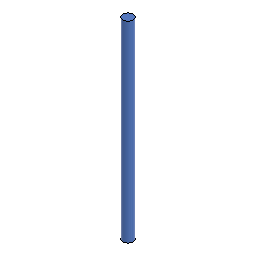
Final Pure Assembly (Autodesk Fusion 360 archive; units mm, degrees)
design "FPA_Guiding Rod"
Autodesk Fusion 360 part; units mm, degrees
(part 1 of 2)
sketch "Sketch2" plane through (0, 0, 0) normal (0, 0, 1) x (1, 0, 0)
  circle A0 centre (0, 0) radius 4
  dimension "d2" = 8
  constraint coincident A0.centre origin
  measures "d2" diameter of A0
extrude "Extrude1" add sketch "Sketch2" along normal blind 150 in component "8mm Diameter Guiding Rod"
component "8mm Diameter Guiding Rod" placed x (1, 0, 0) y (0, 1, 0) z (0, 0, 1) at (0, 0, 0)
equation "length = 150 mm"
equation "d4 = length"

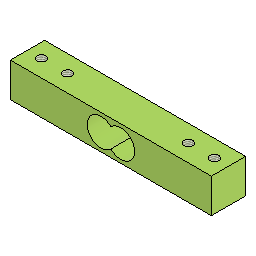
design "FPA_Load Cell"
Autodesk Fusion 360 part; units mm, degrees
sketch "Sketch1" plane through (0, 0, 0) normal (1, 0, 0) x (0, 1, 0)
  line L0 (0, 0) -> (12.8, 0)
  line L1 (12.8, 0) -> (12.8, 12.8)
  line L2 (12.8, 12.8) -> (0, 12.8)
  line L3 (0, 12.8) -> (0, 0)
  dimension "d1" = 12.8
  dimension "d2" = 12.8
  constraint horizontal L0
  constraint vertical L1
  constraint horizontal L2
  constraint vertical L3
  constraint coincident L0.start L3.end
  measures "d1" distance of L0.start L0.end
  measures "d2" distance of L0.start L2.end
extrude "Extrude1" add sketch "Sketch1" along normal blind 75.1 in component "Load Cell"
sketch "Sketch2" plane through (0, 0, 0) normal (0, -1, 0) x (1, 0, 0)
  line L0 (0, 12.8) -> (0, 0)
  line L1 (0, 0) -> (75.1, 0)
  line L2 (75.1, 0) -> (75.1, 12.8)
  line L3 (75.1, 12.8) -> (0, 12.8)
  line L4 (0, 6.4) -> (75.1, 6.4) construction
  line L5 (75.1, 6.4) -> (46.4, 6.4) construction
  circle A0 centre (41.25, 6.4) radius 5.15
  line L6 (37.55, 0) -> (37.55, 12.8) construction
  circle A1 centre (33.85, 6.4) radius 5.15
  point P0 (37.55, 9.9822)
  point P1 (37.55, 2.8178)
  point P2 (28.7, 6.4)
  dimension "d5" = 28.7
  dimension "d6" = 10.3
  dimension "d7" = 7.1645
  dimension "d8" = 28.7
  constraint midpoint L0 L4.start
  constraint midpoint L2 L4.end
  constraint coincident L4 L5.end
  constraint coincident L4 A0.centre
  constraint coincident L5.end A0
  constraint midpoint L1 L6.start
  constraint midpoint L3 L6.end
  constraint symmetric A0 L6 A1
  constraint coincident L6 P0
  constraint coincident A1 P0
  constraint coincident A1 P1
  constraint coincident A0 P1
  constraint coincident A1 P2
  constraint coincident L4 P2
  measures "d5" distance of L4.end L5.end
  measures "d6" diameter of A0
  measures "d7" distance of P0 P1
  measures "d8" distance of L4.start P2
extrude "Extrude2" cut sketch "Sketch2" against normal blind 12.8 contours A0 A1 | A0 A1 | A0 A1 in component "Load Cell"
sketch "Sketch3" plane through (0, 0, 12.8) normal (0, 0, 1) x (-1, 0, 0)
  line L0 (0, -12.8) -> (0, 0)
  line L1 (0, 0) -> (-75.1, 0)
  line L2 (-75.1, 0) -> (-75.1, -12.8)
  line L3 (-75.1, -12.8) -> (0, -12.8)
  line L4 (-75.1, -6.4) -> (0, -6.4) construction
  line L5 (-75.1, -6.4) -> (-71.5, -6.4) construction
  circle A0 centre (-69.834, -6.4) radius 1.666
  circle A1 centre (-60.102, -6.4) radius 1.666
  line L6 (-37.55, -12.8) -> (-37.55, 0) construction
  circle A2 centre (-14.998, -6.4) radius 1.666
  circle A3 centre (-5.266, -6.4) radius 1.666
  point P0 (-71.5, -6.4)
  point P1 (-61.768, -6.4)
  point P2 (-68.168, -6.4)
  dimension "d11" = 3.6
  dimension "d25" = 3.332
  dimension "d26" = 6.4
  constraint midpoint L2 L4.start
  constraint midpoint L0 L4.end
  constraint perpendicular L2 L5
  constraint coincident L4 A0.centre
  constraint coincident A0 P0
  constraint coincident L4 P0
  constraint coincident P0 L5.end
  constraint coincident L4 A1.centre
  constraint equal A0 A1
  constraint coincident A1 P1
  constraint coincident L4 P1
  constraint coincident A0 P2
  constraint coincident L4 P2
  constraint midpoint L3 L6.start
  constraint midpoint L1 L6.end
  constraint symmetric A0 L6 A3
  constraint symmetric A1 L6 A2
  measures "d11" distance of L4.start P0
  measures "d25" diameter of A0
  measures "d26" distance of P1 P2
hole "Hole3" at (5.266, 6.4, 12.8) at (14.998, 6.4, 12.8) at (60.102, 6.4, 12.8) at (69.834, 6.4, 12.8) direction (0, 0, -1) diameter 3.332 depth 16 tip angle 118 in component "Load Cell"
thread "Thread3" "ISO Metric profile 4.0 M4x0.7 M4x0.7 6H" thread offset 0 thread depth 7.4 in component "Load Cell"
component "Load Cell" placed x (1, 0, 0) y (0, 1, 0) z (0, 0, 1) at (0, 0, 0)

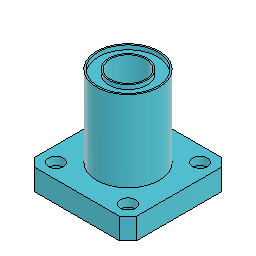
design "FPA_ Linear Bearing Square Flange"
Autodesk Fusion 360 part; units mm, degrees
sketch "Sketch1" plane through (0, 0, 0) normal (0, 0, 1) x (1, 0, 0)
  circle A0 centre (0, 0) radius 4
  circle A1 centre (0, 0) radius 7.5
  line L0 (12, -12) -> (-12, -12)
  line L1 (-12, -12) -> (-12, 12)
  line L2 (-12, 12) -> (12, 12)
  line L3 (12, 12) -> (12, -12)
  line L4 (12, -12) -> (-12, 12) construction
  line L5 (-12, -12) -> (12, 12) construction
  circle A2 centre (0, 0) radius 12 construction
  circle A3 centre (8.4853, 8.4853) radius 1.75
  circle A4 centre (8.4853, 8.4853) radius 3
  circle A5 centre (-8.4853, 8.4853) radius 3
  circle A6 centre (-8.4853, 8.4853) radius 1.75
  circle A7 centre (-8.4853, -8.4853) radius 3
  circle A8 centre (-8.4853, -8.4853) radius 1.75
  circle A9 centre (8.4853, -8.4853) radius 3
  circle A10 centre (8.4853, -8.4853) radius 1.75
  dimension "d1" = 8
  dimension "d2" = 15
  dimension "d3" = 24
  dimension "d4" = 24
  dimension "d5" = 24
  dimension "d8" = 3.5
  dimension "d9" = 6
  dimension "d11" = 360
  constraint coincident A0.centre A1.centre
  constraint horizontal L0
  constraint perpendicular L0 L1
  constraint parallel L0 L2
  constraint parallel L1 L3
  constraint coincident L4 A0.centre
  constraint coincident L5 A0.centre
  constraint concentric A0 A2
  constraint coincident L5 A3.centre
  constraint coincident A2 A3.centre
  constraint concentric A3 A4
  measures "d1" diameter of A0
  measures "d2" diameter of A1
  measures "d3" distance of L1.end L2.end
  measures "d4" distance of L0.end L1.end
  measures "d5" diameter of A2
  measures "d8" diameter of A3
  measures "d9" diameter of A4
extrude "Extrude1" add sketch "Sketch1" against normal blind 5 contours A0 | A1 | L0 L1 L2 L3 | A3 | A4 | A5 | A6 | A7 | A8 | A9 | A10 in component "Component"
extrude "Extrude2" cut sketch "Sketch1" against normal blind 1.9 contours A3 | A6 | A8 | A10 in component "Component"
sketch "Sketch2" plane through (0, 0, -5) normal (0, 0, -1) x (1, 0, 0)
  line L0 (-12, -12) -> (12, -12)
  line L1 (12, -12) -> (12, 12)
  line L2 (12, 12) -> (-12, 12)
  line L3 (-12, 12) -> (-12, -12)
  circle A0 centre (8.4853, 8.4853) radius 3
  circle A1 centre (8.4853, -8.4853) radius 3
  circle A2 centre (-8.4853, -8.4853) radius 3
  circle A3 centre (-8.4853, 8.4853) radius 3
extrude "Extrude3" cut sketch "Sketch2" against normal blind 3.1 contours A0 | A1 | A2 | A3 in component "Component"
extrude "Extrude4" add sketch "Sketch1" along normal blind 19 contours A1 in component "Component"
sketch "Sketch3" plane through (0, 0, 19) normal (0, 0, 1) x (-1, 0, 0)
  circle A0 centre (0, 0) radius 4
  circle A1 centre (0, 0) radius 7.5
  circle A2 centre (0, 0) radius 4
  circle A3 centre (0, 0) radius 7.5
  circle A4 centre (0, 0) radius 4.5
  circle A5 centre (0, 0) radius 7
  dimension "d18" = 0.5
  dimension "d19" = -0.5
extrude "Extrude5" cut sketch "Sketch3" against normal blind 1 contours A5 in component "Component"
extrude "Extrude6" cut 1 faces at (-1.2456, 0.0132, 0) along direction (0, 0, -1) blind 5 in component "Component"
sketch "Sketch4" plane through (0, 0, -5) normal (0, 0, -1) x (1, 0, 0)
  line L0 (12, -12) -> (12, 12)
  line L1 (12, 12) -> (-12, 12)
  line L2 (-12, 12) -> (-12, -12)
  line L3 (-12, -12) -> (12, -12)
  circle A0 centre (0, 0) radius 4
  circle A1 centre (-8.4853, -8.4853) radius 3
  circle A2 centre (8.4853, -8.4853) radius 3
  circle A3 centre (-8.4853, 8.4853) radius 3
  circle A4 centre (8.4853, 8.4853) radius 3
  circle A5 centre (0, 0) radius 4.5
  circle A6 centre (0, 0) radius 4
  circle A7 centre (0, 0) radius 7
  circle A8 centre (0, 0) radius 7.5
extrude "Extrude7" cut sketch "Sketch4" against normal blind 1 contours A7 in component "Component"
move_face "OffsetFaces1" offset -0.15 1 faces at (3.995, -0.1994, 11) in component "Component"
chamfer "Chamfer2" distance 2 angle 45 4 edges at (-12, -12, -2.5) (-12, 12, -2.5) (12, -12, -2.5) (12, 12, -2.5) in component "Component"
move_face "OffsetFaces2" offset -0.15 1 faces at (7.4907, 0.3738, 6.3333) in component "Component"
component "Component" placed x (1, 0, 0) y (0, 1, 0) z (0, 0, 1) at (0, 0, 0)

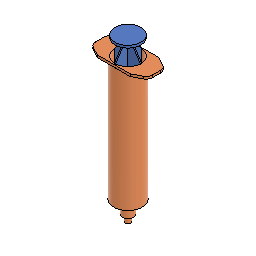
design "FPA_20ml Luer Lock Syringe"
Autodesk Fusion 360 part; units mm, degrees
sketch "Sketch1" plane through (0, 0, 0) normal (0, 1, 0) x (1, 0, 0)
  line L0 (0, 0) -> (11.155, 0)
  line L1 (11.155, 0) -> (11.155, -115) construction
  line L2 (11.155, 0) -> (11.155, -95)
  line L3 (11.155, -95) -> (11.155, -101.75) construction
  line L4 (11.155, -101.75) -> (11.155, -110) construction
  line L5 (11.155, -95) -> (4.4407, -96.7991)
  line L6 (11.155, -95) -> (0, -95) construction
  line L7 (4.4407, -96.7991) -> (4.4407, -105.0848)
  line L8 (4.4407, -105.0848) -> (2.2202, -105.0848)
  line L9 (2.2202, -105.0848) -> (2.2202, -110.0848)
  line L10 (0, -110.0848) -> (2.2202, -110.0848)
  line L11 (0, 0) -> (0, -110.0848)
  dimension "d1" = 11.155
  dimension "d3" = 95
  dimension "d4" = 6.75
  dimension "d5" = 8.25
  dimension "d6" = 165
  dimension "d7" = 2.2205
  dimension "d8" = 8.2857
  dimension "d9" = 5
  dimension "d10" = 2.2202
  dimension "d66" = 115
  dimension "d67" = 110.0848
  constraint coincident L0.start L11.start
  constraint horizontal L0
  constraint perpendicular L0 L1
  constraint perpendicular L0 L2
  constraint parallel L1 L3
  constraint parallel L1 L4
  constraint horizontal L6
  constraint parallel L4 L7
  constraint perpendicular L1 L8
  constraint perpendicular L8 L9
  constraint vertical L11
  constraint perpendicular L10 L11
  constraint coincident L6.end L11
  measures "d1" distance of L0.start L0.end
  measures "d3" distance of L0.end L2.end
  measures "d4" distance of L2.end L3.end
  measures "d5" distance of L3.end L4.end
  measures "d6" angle of L5 L6
  measures "d7" distance of L7.end L8.end
  measures "d8" distance of L5.end L7.end
  measures "d9" distance of L8.end L9.end
  measures "d10" distance of L9.end L10.start
  measures "d66" distance of L0.end L1.end
  measures "d67" distance of L0.start L10.start
revolve "Revolve1" add sketch "Sketch1" angle 360 about axis through (0, 0, 0) along (0, 0, 1) makes body 1 in component "30ml Luer Lock Barrel"
shell "Shell1" thickness 1 removed faces 1 at (-1.6561, 2.7028, 0) on bodies 1 in component "30ml Luer Lock Barrel"
sketch "Sketch2" plane through (0, 0, 110.0848) normal (0, 0, 1) x (-1, 0, 0)
  circle A0 centre (0, 0) radius 2.2202
  circle A1 centre (0, 0) radius 1.2202
extrude "Extrude1" cut sketch "Sketch2" against normal blind 6.86 contours A1 bodies 1 in component "30ml Luer Lock Barrel"
sketch "Sketch3" plane through (0, 0, 0) normal (0, 0, -1) x (1, 0, 0)
  circle A0 centre (0, 0) radius 10.155
  circle A1 centre (0, 0) radius 11.155
  line L0 (22.35, -11.155) -> (-22.35, -11.155)
  line L1 (-22.35, -11.155) -> (-22.35, 11.155)
  line L2 (-22.35, 11.155) -> (22.35, 11.155)
  line L3 (22.35, 11.155) -> (22.35, -11.155)
  line L4 (22.35, -11.155) -> (-22.35, 11.155) construction
  line L5 (-22.35, -11.155) -> (22.35, 11.155) construction
  circle A2 centre (0, 0) radius 10.155
  dimension "d15" = 44.7
  dimension "d16" = 22.31
  constraint horizontal L0
  constraint perpendicular L0 L1
  constraint parallel L0 L2
  constraint parallel L1 L3
  constraint coincident L4 A0.centre
  constraint coincident L5 A0.centre
  constraint coincident A0.centre A1.centre
  measures "d15" distance of L1.end L2.end
  measures "d16" distance of L0.end L1.end
extrude "Extrude2" add sketch "Sketch3" along normal blind 1.86 bodies 1 in component "30ml Luer Lock Barrel"
chamfer "Chamfer1" distance 5 distance2 9.5 2 edges at (22.35, -11.155, -0.93) (-22.35, 11.155, -0.93) measured on face at (22.35, -3.7183, -0.62) measured on face at (-22.35, 3.7183, -0.62) tangent chain off on bodies 1 in component "30ml Luer Lock Barrel"
chamfer "Chamfer1" distance 9.5 distance2 5 2 edges at (22.35, 11.155, -0.93) (-22.35, -11.155, -0.93) measured on face at (0, 11.155, -1.24) measured on face at (0, -11.155, -1.24) tangent chain off on bodies 1 in component "30ml Luer Lock Barrel"
fillet "Fillet1" radius 5 4 edges at (22.35, -6.155, -0.93) (22.35, 6.155, -0.93) (-22.35, -6.155, -0.93) (-22.35, 6.155, -0.93) on bodies 1 in component "30ml Luer Lock Barrel"
sketch "Sketch4" plane through (0, 0, 0) normal (0, 1, 0) x (1, 0, 0)
  line L0 (-11.155, -95) -> (11.155, -95)
  line L1 (-4.4407, -96.7991) -> (4.4407, -96.7991)
  line L2 (-4.4407, -96.7991) -> (-11.155, -95)
  line L3 (-11.155, -95) -> (11.155, -95)
  line L4 (11.155, -95) -> (4.4407, -96.7991)
  line L5 (-4.4407, -96.7991) -> (0, -97.989)
  line L6 (0, -97.989) -> (4.4407, -96.7991)
  line L7 (0, -96.9537) -> (3.5592, -96)
  line L8 (-3.5592, -96) -> (0, -96.9537)
  line L9 (-3.5592, -96) -> (3.5592, -96) construction
  line L10 (-3.5592, -96) -> (-7.2913, -95)
  line L11 (-7.2913, -95) -> (7.2913, -95)
  line L12 (-10.155, -94.2327) -> (10.155, -94.2327)
  line L13 (0, -96.9537) -> (0, -94.2327)
  line L14 (-10.155, -94.2327) -> (10.155, -94.2327)
  line L15 (-3.4407, -96.0318) -> (3.4407, -96.0318)
  line L16 (3.5592, -96) -> (10.155, -94.2327)
  dimension "d68" = 1
  constraint coincident L1.start L2.start
  constraint coincident L0.start L2.end
  constraint coincident L0.end L3.end
  constraint coincident L1.end L4.end
  constraint parallel L2 L5
  constraint parallel L4 L6
  constraint coincident L0 L10.end
  constraint parallel L8 L10
  constraint coincident L0 L11.end
  constraint midpoint L12 L13.end
  constraint coincident L12.end L14.end
  constraint coincident L11.end L16
revolve "Revolve1'" add sketch "Sketch4" angle 360 about axis through (0, 0, 1.75) along (0, 0, 1) separate body contours L0 L3 L11 L12 L13 L14 L16 | L0 L3 L7 L11 L13 L15 L16 | L1 L7 L13 L15 makes body 2 in component "30ml Luer Lock Plunger"
sketch "Sketch5" plane through (0, 0, 94.2327) normal (0, 0, -1) x (1, 0, 0)
  circle A0 centre (0, 0) radius 10.155
  circle A1 centre (0, 0) radius 7.2913
  circle A2 centre (0, 0) radius 10.155
extrude "Extrude1'" add sketch "Sketch5" along normal blind 5 contours A0 A2 | A1 bodies 2 in component "30ml Luer Lock Plunger"
sketch "Sketch6" plane through (0, 0, 89.2327) normal (0, 0, -1) x (1, 0, 0)
  circle A0 centre (0, 0) radius 10.155
  line L0 (0, 0) -> (10.155, 0) construction
  line L1 (0, 0) -> (0, 10.155) construction
  line L2 (-0.5, 0) -> (-0.5, 10.1427)
  line L3 (0.5, 0) -> (0.5, 10.1427)
  line L4 (0, 0) -> (-10.155, 0) construction
  line L5 (-0.5, 0) -> (0.5, 0)
  dimension "d31" = 0.5
  constraint coincident A0.centre L0.start
  constraint coincident A0 L0.end
  constraint horizontal L0
  constraint coincident A0 L1.end
  constraint perpendicular L0 L1
  constraint coincident A0 L3.end
  constraint coincident A0 L2.end
  constraint coincident A0 L4.end
  constraint perpendicular L1 L4
  constraint coincident L2.start L4
  constraint coincident L0 L3.start
extrude "Extrude1''" add sketch "Sketch6" along normal blind 91.446 separate body contours A0 L2 L3 L5 picked at (-0.0556, 3.3845) makes body 3
extrude "Extrude2'" add 1 faces at (-0.0556, -3.3845, -2.2133) along direction (0, 0, -1) blind 14.1 on bodies 3 bodies 3
sketch "Sketch7" plane through (0.5, 0, 0) normal (1, 0, 0) x (0, 1, 0)
  line L0 (0, 89.2327) -> (-10.1427, 89.2327)
  line L1 (-10.1427, 89.2327) -> (-10.1427, -16.3133)
  line L2 (-10.1427, -16.3133) -> (0, -16.3133)
  line L3 (0, -16.3133) -> (0, 89.2327)
  line L4 (0, -16.3133) -> (-10.1427, -16.3133)
  line L5 (0, -16.3133) -> (-5.0713, -16.3133)
  line L6 (-10.1427, -16.3133) -> (-2.5357, -16.3133)
  line L7 (-6.3392, -16.3133) -> (-3.4713, -12.2176)
  line L8 (-6.3392, -16.3133) -> (0, -16.3133) construction
  line L9 (-11.155, -1.86) -> (-7.5609, -1.86)
  line L10 (-3.4713, -12.2176) -> (-10.1427, -1.86)
  line L11 (-11.155, -1.86) -> (-11.155, -0.2883)
  line L12 (-10.1427, -1.86) -> (-11.155, -0.2883)
  line L13 (-11.155, -1.86) -> (-11.155, -16.3133)
  line L14 (-11.155, -16.3133) -> (-10.1427, -16.3133)
  dimension "d37" = 5
  dimension "d38" = 55
  constraint coincident L2.end L3.start
  constraint coincident L1.end L2.start
  constraint midpoint L4 L5.end
  constraint midpoint L5 L6.end
  constraint horizontal L8
  constraint midpoint L6 L7.start
  constraint coincident L9 L10.end
  constraint coincident L1 L10.end
  constraint coincident L9.start L11.start
  constraint perpendicular L9 L11
  constraint parallel L10 L12
  constraint coincident L11.end L12.end
  constraint perpendicular L4 L13
  constraint perpendicular L1 L14
  measures "d37" distance of L7.start L7.end
  measures "d38" angle of L7 L8
extrude "Extrude3" cut sketch "Sketch7" against normal blind 1 contours L1 L2 L4 L6 L7 L10 | L1 L9 L13 L14 bodies 3
fillet "Fillet1'" radius 2.5 1 edges at (0, -3.4713, -12.2176) on bodies 3
pattern_circular "C-Pattern1" count 4 over 360 about axis through (0, 0, 1.75) along (0, 0, 1) of bodies 3 makes body 4 at (6.7618, 0.5, 58.8684) makes body 5 at (-0.5, 6.7618, 58.8684) makes body 6 at (-6.7618, -0.5, 58.8684)
sketch "Sketch8" plane through (0, 0, -16.3133) normal (0, 0, -1) x (1, 0, 0)
  line L0 (0.5, 6.3392) -> (-0.5, 6.3392)
  line L1 (-0.5, 6.3392) -> (-0.5, 0)
  line L2 (-0.5, 0) -> (0.5, 0)
  line L3 (0.5, 0) -> (0.5, 6.3392)
  arc A0 (-22.35, -3.1363) -> (-19.6787, -7.5609) centre (-17.35, -3.1363) ccw
  line L4 (-19.6787, -7.5609) -> (-12.85, -11.155)
  line L5 (-12.85, -11.155) -> (12.85, -11.155)
  line L6 (12.85, -11.155) -> (19.6787, -7.5609)
  arc A1 (19.6787, -7.5609) -> (22.35, -3.1363) centre (17.35, -3.1363) ccw
  line L7 (22.35, -3.1363) -> (22.35, 3.1363)
  arc A2 (22.35, 3.1363) -> (19.6787, 7.5609) centre (17.35, 3.1363) ccw
  line L8 (19.6787, 7.5609) -> (12.85, 11.155)
  line L9 (12.85, 11.155) -> (-12.85, 11.155)
  line L10 (-12.85, 11.155) -> (-19.6787, 7.5609)
  arc A3 (-19.6787, 7.5609) -> (-22.35, 3.1363) centre (-17.35, 3.1363) ccw
  line L11 (-22.35, 3.1363) -> (-22.35, -3.1363)
  circle A4 centre (0, 0) radius 10.155
  circle A5 centre (0, 0) radius 10.155
  dimension "d47" = 20.31
  constraint concentric A4 A5
  measures "d47" diameter of A5
extrude "Extrude4" add sketch "Sketch8" against normal blind 1.86 separate body contours L0 L1 L2 L3 | A4 A5 makes body 7
combine "Combine1" operation add target body 2 tool bodies 4 7 3 6 5 in component "30ml Luer Lock Plunger"
move_body "Move1" bodies 2 to x (-1, 0, 0) y (0, 1, 0) z (0, 0, -1) at (0, 0, 115) in component "30ml Luer Lock Plunger"
move_body "Move1'" bodies 1 to x (-1, 0, 0) y (0, 1, 0) z (0, 0, -1) at (0, 0, 115) in component "30ml Luer Lock Barrel"
component "30ml Luer Lock Barrel" placed x (1, 0, 0) y (0, 1, 0) z (0, 0, 1) at (0, 0, 0)
component "30ml Luer Lock Plunger" placed x (1, 0, 0) y (0, 1, 0) z (0, 0, 1) at (0, 0, 0)
equation "d1 = InnerDiameter"
equation "d4 = 4.5 * 1.5 mm"
equation "d5 = 5.5 * 1.5 mm"
equation "d7 = ( 4.441 / 2 ) * 1 mm"
equation "InnerDiameter = 11.155 mm"
equation "d30 = -offset"
equation "d31 = offset"
equation "offset = 0.5 mm"

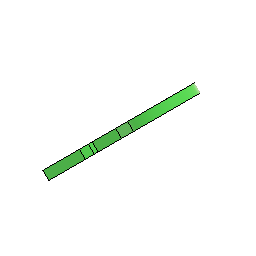
design "FPA_Push Plate Top"
Autodesk Fusion 360 part; units mm, degrees
sketch "sketch 340" plane through (-162.9161, 0, 162.9161) normal (-0.707107, 0, 0.707107) x (0, -1, 0)
  circle A0 centre (-48.0451, 12.2432) radius 1.75
  circle A1 centre (-62.1873, -10.4147) radius 1.75
  line L0 (-62.568, 0) -> (-62.568, -6.4)
  line L1 (-62.568, -6.4) -> (-63.702, -6.9)
  line L2 (-63.702, -6.9) -> (-65.702, -8.9)
  line L3 (-65.702, -8.9) -> (-65.702, -28.9)
  line L4 (-65.702, -28.9) -> (-63.702, -30.9)
  line L5 (-63.702, -30.9) -> (-43.702, -30.9)
  line L6 (-43.702, -30.9) -> (-41.702, -28.9)
  line L7 (-41.702, -28.9) -> (-41.702, -8.9)
  line L8 (-41.702, -8.9) -> (-43.702, -6.9)
  line L9 (-44.836, -6.4) -> (-43.702, -6.9)
  line L10 (-44.836, 0) -> (-44.836, -6.4)
  line L11 (-44.836, 0) -> (-44.836, 6.4)
  line L12 (-44.836, 6.4) -> (-42.9272, 15.6851)
  arc A2 (-42.9272, 15.6851) -> (-64.4766, 15.6852) centre (-53.7019, 17.9) ccw
  arc A3 (-42.9272, 15.6851) -> (-64.4766, 15.6852) centre (-53.7019, 17.9) ccw
  line L13 (-62.568, 6.4) -> (-64.4766, 15.6852)
  line L14 (-62.568, 0) -> (-62.568, 6.4)
  circle A4 centre (-48.0451, 23.5569) radius 1.75
  circle A5 centre (-53.702, -18.9) radius 7.7
  circle A6 centre (-59.3588, 12.2432) radius 1.75
  circle A7 centre (-45.2167, -10.4147) radius 1.75
  circle A8 centre (-45.2167, -27.3853) radius 1.75
  circle A9 centre (-62.1873, -27.3853) radius 1.75
  circle A10 centre (-48.836, 0) radius 1.666
  circle A11 centre (-59.3588, 23.5569) radius 1.75
  circle A12 centre (-58.568, 0) radius 1.666
  circle A13 centre (-53.7019, 17.9) radius 5.3
extrude "Extrude1" add sketch "sketch 340" along normal blind 3.202
sketch "Sketch1" plane through (-165.1802, 0, 165.1802) normal (-0.707107, 0, 0.707107) x (0, -1, 0)
  circle A0 centre (-59.3588, 23.5569) radius 1.75
  circle A1 centre (-45.2167, -10.4147) radius 1.75
  line L0 (-62.568, -6.4) -> (-63.702, -6.9)
  line L1 (-63.702, -6.9) -> (-65.702, -8.9)
  line L2 (-65.702, -8.9) -> (-65.702, -28.9)
  line L3 (-65.702, -28.9) -> (-63.702, -30.9)
  line L4 (-63.702, -30.9) -> (-43.702, -30.9)
  line L5 (-43.702, -30.9) -> (-41.702, -28.9)
  line L6 (-41.702, -28.9) -> (-41.702, -8.9)
  line L7 (-41.702, -8.9) -> (-43.702, -6.9)
  line L8 (-43.702, -6.9) -> (-44.836, -6.4)
  line L9 (-44.836, -6.4) -> (-44.836, 6.4)
  line L10 (-44.836, 6.4) -> (-42.9272, 15.6851)
  arc A2 (-42.9272, 15.6851) -> (-64.4766, 15.6852) centre (-53.7019, 17.9) ccw
  line L11 (-64.4766, 15.6852) -> (-62.568, 6.4)
  line L12 (-62.568, 6.4) -> (-62.568, -6.4)
  circle A3 centre (-53.702, -18.9) radius 7.7
  circle A4 centre (-48.836, 0) radius 1.666
  circle A5 centre (-45.2167, -27.3853) radius 1.75
  circle A6 centre (-48.0451, 12.2432) radius 1.75
  circle A7 centre (-48.0451, 23.5569) radius 1.75
  circle A8 centre (-59.3588, 12.2432) radius 1.75
  circle A9 centre (-62.1873, -27.3853) radius 1.75
  circle A10 centre (-58.568, 0) radius 1.666
  circle A11 centre (-62.1873, -10.4147) radius 1.75
  circle A12 centre (-53.7019, 17.9) radius 5.3
  circle A13 centre (-48.836, 0) radius 2.25
  circle A14 centre (-58.568, 0) radius 2.25
  dimension "d2" = 4.5
  constraint concentric A4 A13
  constraint concentric A10 A14
  constraint equal A13 A14
  measures "d2" diameter of A13
extrude "Extrude2" cut sketch "Sketch1" against normal blind 3.202 contours A13 | A14
equation "m4 = 4.5 mm"
equation "d2 = m4"
named bodies: "PPTop"

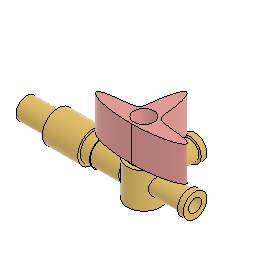
design "FPA_3 way Stopcock"
Autodesk Fusion 360 part; units mm, degrees
sketch "Sketch1" plane through (0, 0, 0) normal (0, 0, 1) x (1, 0, 0)
  circle A0 centre (0, 0) radius 5.27
  circle A1 centre (0, 0) radius 4
  dimension "d1" = 10.54
  dimension "d4" = 8
  constraint coincident A0.centre A1.centre
  measures "d1" diameter of A0
  measures "d4" diameter of A1
extrude "Extrude1" add sketch "Sketch1" along normal blind 11.1 makes body 1
sketch "Sketch2" plane through (0, 0, 0) normal (1, 0, 0) x (0, 1, 0)
  circle A0 centre (0, 6) radius 3
  circle A1 centre (0, 6) radius 2.05
  line L0 (5.27, 0) -> (-5.27, 0)
  dimension "d5" = 6
  dimension "d6" = 4.1
  dimension "d17" = 6
  constraint concentric A0 A1
  measures "d5" diameter of A0
  measures "d6" diameter of A1
  measures "d17" distance of A0.centre L0
extrude "Extrude2" add sketch "Sketch2" along normal blind 11.2 from surface at 5 separate body makes body 2
extrude "Extrude3" cut sketch "Sketch2" along normal blind 7 and the other way blind 7 contours A1 bodies 1
sketch "Sketch3" plane through (0, 0, 0) normal (0, 1, 0) x (1, 0, 0)
  circle A0 centre (0, -6) radius 2.05
  line L0 (-5.27, 0) -> (5.27, 0)
  dimension "d14" = 4.1
  dimension "d18" = 6
  measures "d14" diameter of A0
  measures "d18" distance of A0.centre L0
extrude "Extrude4" cut sketch "Sketch3" along normal blind 6 bodies 1
copy_body "CopyPasteBodies1" bodies 2 makes body 3
move_body "Move1" bodies 3 to x (0, 1, 0) y (-1, 0, 0) z (0, 0, 1) at (0, 0, 0)
extrude "Extrude5" add 1 faces at (5, 2.6722, 5.851) along direction (-1, 0, 0) blind 1 on bodies 2 bodies 1 3 2
extrude "Extrude6" add 1 faces at (-2.6645, 5, 5.7491) along direction (0, -1, 0) blind 1 on bodies 3 bodies 1 3
sketch "Sketch4" plane through (0, 0, 0) normal (1, 0, 0) x (0, 1, 0)
  circle A0 centre (0, 6) radius 4
  dimension "d23" = 8
  measures "d23" diameter of A0
extrude "Extrude7" add sketch "Sketch4" against normal blind 9 from surface at -4 bodies 1
sketch "Sketch5" plane through (-13, 0, 0) normal (-1, 0, 0) x (0, -1, 0)
  circle A0 centre (0, 6) radius 4
  circle A1 centre (0, 6) radius 4.25
  dimension "d27" = 0.25
extrude "Extrude8" add sketch "Sketch5" along normal blind 3 contours A0 | A1 bodies 1
sketch "Sketch6" plane through (-16, 0, 0) normal (-1, 0, 0) x (0, -1, 0)
  circle A0 centre (0, 6) radius 4.25
  circle A1 centre (0, 6) radius 5
  dimension "d30" = 0.75
extrude "Extrude9" add sketch "Sketch6" along normal blind 11.25 contours A0 | A1 bodies 1
sketch "Sketch7" plane through (-27.25, 0, 0) normal (-1, 0, 0) x (0, -1, 0)
  circle A0 centre (0, 6) radius 5
  circle A1 centre (0, 6) radius 3.35
  dimension "d33" = 6.7
  constraint concentric A0 A1
  measures "d33" diameter of A1
extrude "Extrude10" add sketch "Sketch7" along normal blind 10 contours A1 bodies 1
sketch "Sketch8" plane through (16.2, 0, 0) normal (1, 0, 0) x (0, 1, 0)
  circle A0 centre (0, 6) radius 2.05
  circle A1 centre (0, 6) radius 3
  circle A2 centre (0, 6) radius 3.75
  dimension "d36" = 0.75
extrude "Extrude11" add sketch "Sketch8" against normal blind 1.8 contours A2 bodies 1
sketch "Sketch9" plane through (0, 16.2, 0) normal (0, 1, 0) x (-1, 0, 0)
  circle A0 centre (0, 6) radius 2.05
  circle A1 centre (0, 6) radius 3
  circle A2 centre (0, 6) radius 3.75
  dimension "d39" = 0.75
extrude "Extrude12" add sketch "Sketch9" against normal blind 1.8 contours A2 bodies 1
sketch "Sketch10" plane through (0, 0, 0) normal (0, 0, 1) x (1, 0, 0)
  line L0 (-1.15, 4.3682) -> (1.15, 4.3682)
  line L1 (1.15, 4.3682) -> (1.15, -4.3867)
  line L2 (1.15, -4.3867) -> (-1.15, -4.3867)
  line L3 (-1.15, -4.3867) -> (-1.15, 4.3682)
  dimension "d42" = 2.3
  dimension "d44" = 1.15
  constraint horizontal L0
  constraint vertical L1
  constraint horizontal L2
  constraint vertical L3
  measures "d42" distance of L0.start L0.end
  measures "d44" distance of origin L3
extrude "Extrude13" add sketch "Sketch10" along normal blind 1 from surface at 2.3 bodies 1
sketch "Sketch11" plane through (0, 0, 3.3) normal (0, 0, 1) x (-1, 0, 0)
  arc A0 (-1.15, -3.8311) -> (1.15, -3.8311) centre (0, 0) ccw
  line L0 (1.15, -3.8311) -> (1.15, 3.8311)
  arc A1 (1.15, 3.8311) -> (-1.15, 3.8311) centre (0, 0) ccw
  line L1 (-1.15, 3.8311) -> (-1.15, -3.8311)
  circle A2 centre (0, 0) radius 3.95
  dimension "d48" = 7.9
  constraint coincident A0.centre A1.centre
  measures "d48" diameter of A2
extrude "Extrude14" add sketch "Sketch11" along normal blind 19 separate body contours L1 A2 | L0 L1 A2 | L0 A2 makes body 4
sketch "Sketch12" plane through (0, 0, 22.3) normal (0, 0, 1) x (-1, 0, 0)
  circle A0 centre (0, 0) radius 3.95
  circle A1 centre (0, 0) radius 3.15
  dimension "d51" = 6.3
  constraint coincident A0.centre A1.centre
  measures "d51" diameter of A1
extrude "Extrude15" cut sketch "Sketch12" against normal blind 11.6 contours A1 bodies 1 4
sketch "Sketch13" plane through (0, 0, 22.3) normal (0, 0, 1) x (-1, 0, 0)
  circle A0 centre (0, 0) radius 3.15
  circle A1 centre (0, 0) radius 3.95
  line L0 (0, 0) -> (-13.5, 0) construction
  line L1 (0, 0) -> (0, -13.5) construction
  line L2 (0, 0) -> (13.5, 0) construction
  spline S0 degree 5 poles (0, 3.95) (0.8774, 3.9534) (2.6328, 3.9236) (5.2265, 3.7687) (8.4393, 3.3573) (11.6656, 2.5984) (13.7966, 1.7229) (14.6395, 0.8643) (14.1583, 0.1346) (12.5045, -0.4004) (10.0841, -0.7529) (7.4539, -1.0032) (5.1765, -1.2699) (3.6392, -1.6883) (2.9966, -2.3821) (2.7951, -3.4471) (2.6564, -4.8957) (2.4428, -6.6605) (2.1063, -8.6043) (1.6738, -10.5301) (1.1669, -12.1844) (0.6041, -13.3084) (0.0053, -13.7018) (-0.6032, -13.2822) (-1.1833, -12.1476) (-1.6945, -10.5096) (-2.1019, -8.6293) (-2.3861, -6.7477) (-2.5499, -5.0317) (-2.6754, -3.59) (-2.9206, -2.475) (-3.6496, -1.6976) (-5.248, -1.2176) (-7.5451, -0.9251) (-10.1548, -0.6864) (-12.5326, -0.3702) (-14.1434, 0.1206) (-14.5978, 0.8135) (-13.7482, 1.6503) (-11.6271, 2.5226) (-8.419, 3.2955) (-5.2196, 3.7287) (-2.6316, 3.9032) (-0.8774, 3.9466) (0, 3.95) knots 0 0 0 0 0 0 0.025 0.05 0.075 0.1 0.125 0.15 0.175 0.2 0.225 0.25 0.275 0.3 0.325 0.35 0.375 0.4 0.425 0.45 0.475 0.5 0.525 0.55 0.575 0.6 0.625 0.65 0.675 0.7 0.725 0.75 0.775 0.8 0.825 0.85 0.875 0.9 0.925 0.95 0.975 1 1 1 1 1 1
  line L3 (4.2774, -0.7951) -> (2.169, -3.7715)
  line L4 (-2, -4) -> (-4.3181, -0.7426)
  point P0 (3.2232, -2.2833)
  point P1 (2, -9)
  point P2 (-2, -9)
  point P3 (-3.159, -2.3713)
  constraint coincident A0.centre A1.centre
  constraint horizontal L0
  constraint perpendicular L0 L1
  constraint perpendicular L1 L2
  constraint coincident A1 S0.start
  constraint coincident A1 P0
  constraint coincident A1 P3
  constraint midpoint P0 L3
  constraint tangent A1 L3
  constraint midpoint P3 L4
extrude "Extrude16" add sketch "Sketch13" against normal blind 11 bodies 4
sketch "Sketch14" plane through (0, 0, 0) normal (1, 0, 0) x (0, 1, 0)
  circle A0 centre (0, 6) radius 1
  dimension "d57" = 2
  dimension "d58" = 6
  measures "d57" diameter of A0
  measures "d58" distance of origin A0.centre
extrude "Extrude17" cut sketch "Sketch14" along normal blind 8 and the other way blind 8 bodies 1 4
sketch "Sketch15" plane through (0, 0, 0) normal (0, 1, 0) x (1, 0, 0)
  circle A0 centre (0, -6) radius 1
  dimension "d63" = 2
  dimension "d64" = 6
  measures "d63" diameter of A0
  measures "d64" distance of origin A0.centre
extrude "Extrude18" cut sketch "Sketch15" along normal blind 8 bodies 4
copy_body "Body->Comp1" bodies 4 removing the originals makes body 5 in component "Top"
copy_body "Body->Comp2" bodies 1 removing the originals makes body 6 in component "Bottom"
component "Top" placed x (1, 0, 0) y (0, 1, 0) z (0, 0, 1) at (0, 0, 0)
component "Bottom" placed x (1, 0, 0) y (0, 1, 0) z (0, 0, 1) at (0, 0, 0)
equation "d30 = ( ( 10 - 8.5 ) / 2 ) * 1 mm"
equation "d44 = ( 2.3 / 2 ) * 1 mm"
named bodies: "Bottom", "Top"

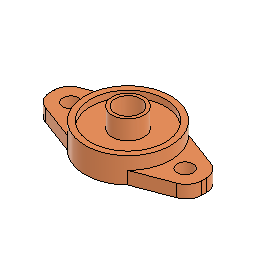
design "FPA_Flange Pillow Block 2"
Autodesk Fusion 360 part; units mm, degrees
sketch "Sketch1" plane through (0, 0, 0) normal (0, 0, 1) x (1, 0, 0)
  line L0 (0, 0) -> (48, 0) construction
  circle A0 centre (24, 0) radius 13.5
  line L1 (24, 0) -> (42, 0) construction
  circle A1 centre (42, 0) radius 2.5
  line L2 (24, 0) -> (24, -13.5) construction
  circle A2 centre (6, 0) radius 2.5
  line L3 (42, 0) -> (42, -6.4) construction
  line L4 (33.4916, 0) -> (33.4916, -9.6) construction
  line L5 (33.4916, -9.6) -> (42, -6.4)
  line L6 (48, 0) -> (48, -0.682)
  line L7 (44.7601, -5.3619) -> (42, -6.4)
  arc A3 (44.7601, -5.3619) -> (48, -0.682) centre (43, -0.682) ccw
  line L8 (33.4916, 9.6) -> (42, 6.4)
  line L9 (44.7601, 5.3619) -> (42, 6.4)
  arc A4 (48, 0.682) -> (44.7601, 5.3619) centre (43, 0.682) ccw
  line L10 (48, 0) -> (48, 0.682)
  line L11 (14.5084, 9.6) -> (6, 6.4)
  line L12 (3.2399, 5.3619) -> (6, 6.4)
  arc A5 (3.2399, 5.3619) -> (0, 0.682) centre (5, 0.682) ccw
  arc A6 (0, -0.682) -> (3.2399, -5.3619) centre (5, -0.682) ccw
  line L13 (0, 0) -> (0, 0.682)
  line L14 (0, 0) -> (0, -0.682)
  line L15 (3.2399, -5.3619) -> (6, -6.4)
  line L16 (14.5084, -9.6) -> (6, -6.4)
  circle A7 centre (24, 0) radius 4
  circle A8 centre (24, 0) radius 5
  circle A9 centre (24, 0) radius 11.75
  dimension "d1" = 48
  dimension "d2" = 27
  dimension "d3" = 18
  dimension "d4" = 5
  dimension "d5" = 6.4
  dimension "d6" = 9.6
  dimension "d8" = 5
  dimension "d9" = 8
  dimension "d10" = 10
  dimension "d13" = -1.75
  constraint coincident L0.start L13.start
  constraint horizontal L0
  constraint midpoint L0 A0.centre
  constraint coincident A0.centre L1.start
  constraint parallel L0 L1
  constraint coincident L1.end A1.centre
  constraint coincident A0 L2.end
  constraint perpendicular L0 L2
  constraint symmetric A1 L2 A2
  constraint perpendicular L1 L3
  constraint coincident L1 L4.start
  constraint perpendicular L1 L4
  constraint coincident A0 L4.end
  constraint perpendicular L0 L6
  constraint parallel L5 L7
  constraint tangent L7 A3
  constraint tangent L6 A3
  constraint symmetric L0.end L1 L6.start
  constraint symmetric L1 L3.end L8.end
  constraint symmetric L1 L4.end L8.start
  constraint symmetric L1 L7.start L9.start
  constraint symmetric L1 L6.end A4.start
  constraint symmetric L1 A3 A4
  constraint symmetric L0.end L2 L0.start
  constraint symmetric L2 L3.end L15.end
  constraint symmetric L2 L4.end L16.start
  constraint symmetric L2 L7.start A6.end
  constraint symmetric L2 L6.end A6.start
  constraint symmetric L2 A3 A6
  constraint symmetric L2 L8.start L11.start
  constraint symmetric L2 L8.end L11.end
  constraint symmetric L2 L9.start L12.start
  constraint symmetric L2 A4.start A5.end
  constraint symmetric L2 A4 A5
  constraint symmetric L2 L0.end L0.start
  constraint concentric A0 A7
  constraint concentric A7 A8
  measures "d1" distance of L0.start L0.end
  measures "d2" diameter of A0
  measures "d3" distance of A0.centre L1.end
  measures "d4" diameter of A1
  measures "d5" distance of L1.end L3.end
  measures "d6" distance of L4.start L4.end
  measures "d8" radius of A3
  measures "d9" diameter of A7
  measures "d10" diameter of A8
extrude "Extrude1" add sketch "Sketch1" along normal blind 4 contours A0 | A0 L5 L6 L7 A3 L8 L9 A4 L10 | A0 L11 L12 A5 A6 L13 L14 L15 L16 | A8 | A9 in component "Flange Pillow Block"
sketch "Sketch2" plane through (0, 0, 4) normal (0, 0, 1) x (-1, 0, 0)
  circle A0 centre (-24, 0) radius 4
  circle A1 centre (-6, 0) radius 2.5
  circle A2 centre (-42, 0) radius 2.5
  line L0 (-33.4916, 9.6) -> (-44.7601, 5.3619)
  arc A3 (-44.7601, 5.3619) -> (-48, 0.682) centre (-43, 0.682) ccw
  line L1 (-48, 0.682) -> (-48, -0.682)
  arc A4 (-48, -0.682) -> (-44.7601, -5.3619) centre (-43, -0.682) ccw
  line L2 (-44.7601, -5.3619) -> (-33.4916, -9.6)
  arc A5 (-33.4916, -9.6) -> (-14.5084, -9.6) centre (-24, 0) ccw
  line L3 (-14.5084, -9.6) -> (-3.2399, -5.3619)
  arc A6 (-3.2399, -5.3619) -> (0, -0.682) centre (-5, -0.682) ccw
  line L4 (0, -0.682) -> (0, 0.682)
  arc A7 (0, 0.682) -> (-3.2399, 5.3619) centre (-5, 0.682) ccw
  line L5 (-3.2399, 5.3619) -> (-14.5084, 9.6)
  arc A8 (-14.5084, 9.6) -> (-33.4916, 9.6) centre (-24, 0) ccw
  circle A9 centre (-24, 0) radius 13.5
  circle A10 centre (-24, 0) radius 11.75
  circle A11 centre (-24, 0) radius 5
  circle A12 centre (-24, 0) radius 4
extrude "Extrude2" add sketch "Sketch2" along normal blind 4 contours A5 A8 A9 in component "Flange Pillow Block"
extrude "Extrude3" add sketch "Sketch2" along normal blind 8 contours A11 in component "Flange Pillow Block"
extrude "Extrude4" add 1 faces at (14.5624, 0.8322, 4) along direction (0, 0, 1) blind 2 in component "Flange Pillow Block"
component "Flange Pillow Block" placed x (1, 0, 0) y (0, 1, 0) z (0, 0, 1) at (0, 0, 0)

design "FPA_Lead Screw"
Autodesk Fusion 360 part; units mm, degrees
sketch "Sketch1" plane through (0, 0, 0) normal (0, 0, 1) x (1, 0, 0)
  circle A0 centre (0, 0) radius 4
  dimension "d1" = 8
  constraint coincident A0.centre origin
  measures "d1" diameter of A0
extrude "Extrude1" add sketch "Sketch1" along normal blind 150 makes body 1
thread "Thread1" "ISO Metric Trapezoidal Threads 8.0 TR8x1.5 TR8x1.5 7e" major diameter 7.925 minor diameter 6.0605 pitch 1.5 angle 30 resizes the face on face at (3.995, -0.1994, 100) on bodies 1
copy_body "Body->Comp1" bodies 1 removing the originals makes body 2 in component "T8 Trapezoidal Lead Screw"
chamfer "Chamfer1" distance 0.5 angle 45 2 edges at (-3.6943, -1.4329, 150) (-3.6943, -1.4329, 0) on bodies 2 in component "T8 Trapezoidal Lead Screw"
component "T8 Trapezoidal Lead Screw" placed x (1, 0, 0) y (0, 1, 0) z (0, 0, 1) at (0, 0, 0)
equation "length = 150 mm"
equation "d3 = length"
equation "clearanc = 0.15 mm"

design "FPA_Stepper Support Cap"
Autodesk Fusion 360 part; units mm, degrees
sketch "sketch 809" plane through (0, 74.8519, 0) normal (0, 1, 0) x (-1, 0, 0)
  line L0 (16.2989, 55.9676) -> (29.7339, 69.4027)
  line L1 (29.7339, 69.4027) -> (37.5121, 77.1808)
  line L2 (37.5121, 77.1808) -> (39.0677, 78.7365)
  line L3 (39.0677, 78.7365) -> (33.4109, 84.3933)
  line L4 (29.7339, 88.0703) -> (33.4109, 84.3933)
  line L5 (-29.7339, 88.0703) -> (29.7339, 88.0703)
  line L6 (-29.7339, 88.0703) -> (-33.4109, 84.3933)
  line L7 (-39.0677, 78.7365) -> (-33.4109, 84.3933)
  line L8 (-37.5121, 77.1808) -> (-39.0677, 78.7365)
  line L9 (-29.7339, 69.4027) -> (-37.5121, 77.1808)
  line L10 (-16.2989, 55.9676) -> (-29.7339, 69.4027)
  line L11 (-16.2989, 55.9676) -> (-6.006, 45.6747)
  line L12 (-6.006, 45.6747) -> (6.006, 45.6747)
  line L13 (16.2989, 55.9676) -> (6.006, 45.6747)
extrude "Extrude1" add sketch "sketch 809" along normal blind 2 makes body 1
mirror "Mirror1" about plane through (0, 53.7019, 18.0777) normal (0, -1, 0) of bodies 1 makes body 2
sketch "sketch 862" plane through (0, 74.8519, 0) normal (0, 1, 0) x (-1, 0, 0)
  line L0 (-29.7339, 85.2418) -> (-28.3197, 86.6561)
  line L1 (-28.3197, 86.6561) -> (28.3197, 86.6561)
  line L2 (28.3197, 86.6561) -> (29.7339, 85.2418)
  line L3 (29.7339, 85.2418) -> (31.9966, 82.9791)
  line L4 (37.6535, 77.3223) -> (31.9966, 82.9791)
  line L5 (37.6535, 77.3223) -> (39.0677, 78.7365)
  line L6 (39.0677, 78.7365) -> (33.4109, 84.3933)
  line L7 (29.7339, 88.0703) -> (33.4109, 84.3933)
  line L8 (-29.7339, 88.0703) -> (29.7339, 88.0703)
  line L9 (-29.7339, 88.0703) -> (-33.4109, 84.3933)
  line L10 (-39.0677, 78.7365) -> (-33.4109, 84.3933)
  line L11 (-37.6535, 77.3223) -> (-39.0677, 78.7365)
  line L12 (-37.6535, 77.3223) -> (-31.9966, 82.9791)
  line L13 (-29.7339, 85.2418) -> (-31.9966, 82.9791)
extrude "Extrude3" add sketch "sketch 862" against normal blind 42.3 bodies 1 2
sketch "sketch 913" plane through (-57.3465, 0, 57.3465) normal (-0.707107, 0, 0.707107) x (0, -1, 0)
  circle A0 centre (-38.2019, 33.4) radius 2
  circle A1 centre (-69.2019, 33.4) radius 2
  circle A2 centre (-53.7019, 17.9) radius 12.5
extrude "Extrude4" cut sketch "sketch 913" along normal blind 2.2 bodies 1
mirror "Mirror2" about plane through (0, 0, 0) normal (1, 0, 0) of "Extrude4"
sketch "sketch 934" plane through (0, 30.5519, 0) normal (0, -1, 0) x (1, 0, 0)
  circle A0 centre (0, 51.1747) radius 3
extrude "Extrude5" cut sketch "sketch 934" against normal blind 46.3 bodies 1
sketch "sketch 946" plane through (0, 0, 88.0703) normal (0, 0, 1) x (-1, 0, 0)
  line L0 (-6.4235, -47.7019) -> (-1.8478, -47.7019)
  spline S0 degree 3 poles (-8.3594, -47.9025) (-8.0673, -47.8441) (-7.4287, -47.7164) (-6.7771, -47.707) (-6.4235, -47.7019) knots 0 0 0 0 0.08917 0.194985 0.194985 0.194985 0.194985
  spline S1 degree 3 poles (-9.6732, -48.4959) (-9.4808, -48.3713) (-9.0732, -48.1074) (-8.6061, -47.9733) (-8.3594, -47.9025) knots 0 0 0 0 0.06837 0.144863 0.144863 0.144863 0.144863
  spline S2 degree 3 poles (-10.5531, -49.6133) (-10.4327, -49.3896) (-10.2042, -48.9655) (-9.8437, -48.6467) (-9.6732, -48.4959) knots 0 0 0 0 0.075498 0.14322 0.14322 0.14322 0.14322
  spline S3 degree 3 poles (-10.9092, -51.1808) (-10.895, -50.9061) (-10.8671, -50.3629) (-10.657, -49.8612) (-10.5531, -49.6133) knots 0 0 0 0 0.081829 0.161828 0.161828 0.161828 0.161828
  spline S4 degree 3 poles (-10.3239, -52.998) (-10.4946, -52.7262) (-10.8436, -52.1707) (-10.887, -51.5155) (-10.9092, -51.1808) knots 0 0 0 0 0.09469 0.193596 0.193596 0.193596 0.193596
  spline S5 degree 3 poles (-8.65, -54.0867) (-8.9872, -53.9674) (-9.6339, -53.7388) (-10.1006, -53.2377) (-10.3239, -52.998) knots 0 0 0 0 0.105521 0.20233 0.20233 0.20233 0.20233
  spline S6 degree 3 poles (-9.9106, -55.1835) (-9.748, -54.9652) (-9.4079, -54.5086) (-8.9099, -54.2314) (-8.65, -54.0867) knots 0 0 0 0 0.080705 0.168794 0.168794 0.168794 0.168794
  spline S7 degree 3 poles (-10.328, -56.6324) (-10.31, -56.3786) (-10.2736, -55.8662) (-10.0323, -55.4125) (-9.9106, -55.1835) knots 0 0 0 0 0.075419 0.152276 0.152276 0.152276 0.152276
  spline S8 degree 3 poles (-9.8574, -58.2163) (-9.9946, -57.9638) (-10.2638, -57.4689) (-10.3069, -56.9075) (-10.328, -56.6324) knots 0 0 0 0 0.085121 0.166906 0.166906 0.166906 0.166906
  spline S9 degree 3 poles (-8.5559, -59.3377) (-8.8174, -59.2005) (-9.3381, -58.9274) (-9.6848, -58.4526) (-9.8574, -58.2163) knots 0 0 0 0 0.08733 0.173851 0.173851 0.173851 0.173851
  spline S10 degree 3 poles (-6.3499, -59.7019) (-6.7669, -59.6943) (-7.5212, -59.6805) (-8.2362, -59.4436) (-8.5559, -59.3377) knots 0 0 0 0 0.124243 0.22472 0.22472 0.22472 0.22472
  line L1 (-1.8478, -59.7019) -> (-6.3499, -59.7019)
  line L2 (-1.8478, -47.7019) -> (-1.8478, -59.7019)
  line L3 (-3.4358, -53.2435) -> (-3.4358, -49.118)
  line L4 (-6.2107, -53.2435) -> (-3.4358, -53.2435)
  spline S11 degree 3 poles (-7.9665, -53.043) (-7.7195, -53.1012) (-7.1429, -53.2371) (-6.5498, -53.2412) (-6.2107, -53.2435) knots 0 0 0 0 0.075892 0.177209 0.177209 0.177209 0.177209
  spline S12 degree 3 poles (-8.9201, -52.3472) (-8.7928, -52.5006) (-8.5336, -52.8125) (-8.1577, -52.9653) (-7.9665, -53.043) knots 0 0 0 0 0.058827 0.119686 0.119686 0.119686 0.119686
  spline S13 degree 3 poles (-9.2639, -51.1808) (-9.2513, -51.3947) (-9.2268, -51.8105) (-9.0204, -52.1718) (-8.9201, -52.3472) knots 0 0 0 0 0.063308 0.123078 0.123078 0.123078 0.123078
  spline S14 degree 3 poles (-9.0265, -50.1699) (-9.0957, -50.3247) (-9.2394, -50.6462) (-9.2555, -50.9983) (-9.2639, -51.1808) knots 0 0 0 0 0.050417 0.104665 0.104665 0.104665 0.104665
  spline S15 degree 3 poles (-8.4208, -49.5027) (-8.5394, -49.5903) (-8.7857, -49.7721) (-8.9443, -50.0341) (-9.0265, -50.1699) knots 0 0 0 0 0.043796 0.090887 0.090887 0.090887 0.090887
  spline S16 degree 3 poles (-7.504, -49.1753) (-7.6748, -49.2108) (-7.9958, -49.2775) (-8.2853, -49.4309) (-8.4208, -49.5027) knots 0 0 0 0 0.052017 0.097785 0.097785 0.097785 0.097785
  spline S17 degree 3 poles (-6.4235, -49.118) (-6.6421, -49.1176) (-7.0035, -49.1169) (-7.3623, -49.1588) (-7.504, -49.1753) knots 0 0 0 0 0.0655 0.108281 0.108281 0.108281 0.108281
  line L5 (-3.4358, -49.118) -> (-6.4235, -49.118)
  line L6 (-3.4358, -58.2858) -> (-3.4358, -54.6596)
  line L7 (-5.8342, -58.2858) -> (-3.4358, -58.2858)
  spline S18 degree 3 poles (-7.6595, -58.118) (-7.4194, -58.1665) (-6.8179, -58.2879) (-6.2034, -58.2866) (-5.8342, -58.2858) knots 0 0 0 0 0.073326 0.183705 0.183705 0.183705 0.183705
  spline S19 degree 3 poles (-8.4781, -57.4959) (-8.3715, -57.6357) (-8.1559, -57.9182) (-7.8261, -58.051) (-7.6595, -58.118) knots 0 0 0 0 0.051717 0.104523 0.104523 0.104523 0.104523
  spline S20 degree 3 poles (-8.7646, -56.4441) (-8.7541, -56.635) (-8.7336, -57.0064) (-8.5616, -57.3359) (-8.4781, -57.4959) knots 0 0 0 0 0.056628 0.110142 0.110142 0.110142 0.110142
  spline S21 degree 3 poles (-8.4576, -55.3963) (-8.5471, -55.5494) (-8.736, -55.8725) (-8.7547, -56.247) (-8.7646, -56.4441) knots 0 0 0 0 0.052395 0.110612 0.110612 0.110612 0.110612
  spline S22 degree 3 poles (-7.5449, -54.7988) (-7.7313, -54.8646) (-8.085, -54.9896) (-8.3379, -55.2657) (-8.4576, -55.3963) knots 0 0 0 0 0.058252 0.110587 0.110587 0.110587 0.110587
  spline S23 degree 3 poles (-6.0306, -54.6596) (-6.334, -54.6595) (-6.8437, -54.6591) (-7.3429, -54.7586) (-7.5449, -54.7988) knots 0 0 0 0 0.090722 0.152389 0.152389 0.152389 0.152389
  line L8 (-3.4358, -54.6596) -> (-6.0306, -54.6596)
  spline S24 degree 3 poles (-14.1873, -50.5505) (-13.9868, -51.0296) (-13.5853, -51.9887) (-13.5283, -53.0268) (-13.4998, -53.5464) knots 0 0 0 0 0.154559 0.309405 0.309405 0.309405 0.309405
  spline S25 degree 3 poles (-16.2092, -48.3158) (-15.7912, -48.6139) (-14.954, -49.211) (-14.4431, -50.1036) (-14.1873, -50.5505) knots 0 0 0 0 0.152048 0.304553 0.304553 0.304553 0.304553
  spline S26 degree 3 poles (-19.2378, -47.4973) (-18.6929, -47.5284) (-17.6254, -47.5895) (-16.6746, -48.0771) (-16.2092, -48.3158) knots 0 0 0 0 0.161736 0.316832 0.316832 0.316832 0.316832
  spline S27 degree 3 poles (-22.1519, -48.2381) (-21.6918, -48.022) (-20.768, -47.5882) (-19.7492, -47.5277) (-19.2378, -47.4973) knots 0 0 0 0 0.150977 0.303132 0.303132 0.303132 0.303132
  spline S28 degree 3 poles (-24.2392, -50.4195) (-23.9711, -49.9701) (-23.4418, -49.083) (-22.5781, -48.5173) (-22.1519, -48.2381) knots 0 0 0 0 0.154738 0.305461 0.305461 0.305461 0.305461
  spline S29 degree 3 poles (-24.9759, -53.6856) (-24.9492, -53.1012) (-24.8975, -51.968) (-24.454, -50.9248) (-24.2392, -50.4195) knots 0 0 0 0 0.173897 0.337211 0.337211 0.337211 0.337211
  spline S30 degree 3 poles (-24.276, -56.9066) (-24.4801, -56.4079) (-24.9023, -55.376) (-24.9508, -54.2615) (-24.9759, -53.6856) knots 0 0 0 0 0.160368 0.331829 0.331829 0.331829 0.331829
  spline S31 degree 3 poles (-22.2419, -59.1208) (-22.6608, -58.8288) (-23.503, -58.2418) (-24.0175, -57.3532) (-24.276, -56.9066) knots 0 0 0 0 0.151185 0.303951 0.303951 0.303951 0.303951
  spline S32 degree 3 poles (-19.246, -59.9148) (-19.7821, -59.8841) (-20.8355, -59.8239) (-21.7787, -59.3523) (-22.2419, -59.1208) knots 0 0 0 0 0.159223 0.312844 0.312844 0.312844 0.312844
  spline S33 degree 3 poles (-15.1041, -58.2244) (-15.6875, -58.7174) (-16.8831, -59.7275) (-18.4458, -59.8514) (-19.246, -59.9148) knots 0 0 0 0 0.223252 0.457517 0.457517 0.457517 0.457517
  spline S34 degree 3 poles (-13.4998, -53.5464) (-13.5462, -54.4655) (-13.633, -56.1852) (-14.6368, -57.5766) (-15.1041, -58.2244) knots 0 0 0 0 0.26934 0.504005 0.504005 0.504005 0.504005
  spline S35 degree 3 poles (-16.3524, -57.3895) (-15.9994, -56.8911) (-15.186, -55.7424) (-15.1546, -54.3245) (-15.1369, -53.5218) knots 0 0 0 0 0.179482 0.413625 0.413625 0.413625 0.413625
  spline S36 degree 3 poles (-19.2542, -58.5478) (-18.712, -58.4997) (-17.6288, -58.4038) (-16.7775, -57.7273) (-16.3524, -57.3895) knots 0 0 0 0 0.159505 0.318631 0.318631 0.318631 0.318631
  spline S37 degree 3 poles (-21.3947, -57.9461) (-21.0645, -58.1216) (-20.3949, -58.4774) (-19.6379, -58.5241) (-19.2542, -58.5478) knots 0 0 0 0 0.110798 0.224654 0.224654 0.224654 0.224654
  spline S38 degree 3 poles (-22.8435, -56.2517) (-22.6621, -56.5938) (-22.305, -57.2668) (-21.6948, -57.7222) (-21.3947, -57.9461) knots 0 0 0 0 0.114576 0.225424 0.225424 0.225424 0.225424
  spline S39 degree 3 poles (-23.3388, -53.6937) (-23.3227, -54.1561) (-23.2922, -55.0356) (-22.9879, -55.8605) (-22.8435, -56.2517) knots 0 0 0 0 0.137768 0.262036 0.262036 0.262036 0.262036
  spline S40 degree 3 poles (-22.1805, -50.1167) (-22.5177, -50.6086) (-23.2533, -51.6816) (-23.3087, -52.9869) (-23.3388, -53.6937) knots 0 0 0 0 0.175468 0.382752 0.382752 0.382752 0.382752
  spline S41 degree 3 poles (-19.2296, -48.8561) (-19.7981, -48.9058) (-20.9204, -49.004) (-21.7642, -49.749) (-22.1805, -50.1167) knots 0 0 0 0 0.166415 0.328524 0.328524 0.328524 0.328524
  spline S42 degree 3 poles (-16.3033, -50.1044) (-16.7193, -49.7403) (-17.5583, -49.006) (-18.6694, -48.9063) (-19.2296, -48.8561) knots 0 0 0 0 0.161407 0.325554 0.325554 0.325554 0.325554
  spline S43 degree 3 poles (-15.1369, -53.5218) (-15.1713, -52.8532) (-15.2358, -51.5987) (-15.9635, -50.5801) (-16.3033, -50.1044) knots 0 0 0 0 0.196076 0.36787 0.36787 0.36787 0.36787
  line L9 (11.4576, -47.7019) -> (12.9883, -47.7019)
  line L10 (11.4576, -57.9175) -> (11.4576, -47.7019)
  line L11 (7.987, -47.7019) -> (11.4576, -57.9175)
  line L12 (6.5545, -47.7019) -> (7.987, -47.7019)
  line L13 (3.0675, -57.7456) -> (6.5545, -47.7019)
  line L14 (3.0675, -47.7019) -> (3.0675, -57.7456)
  line L15 (1.5368, -47.7019) -> (3.0675, -47.7019)
  line L16 (1.5368, -59.7019) -> (1.5368, -47.7019)
  line L17 (3.6732, -59.7019) -> (1.5368, -59.7019)
  line L18 (6.5463, -51.3527) -> (3.6732, -59.7019)
  spline S44 degree 3 poles (7.1848, -49.4291) (7.0982, -49.6987) (6.8915, -50.342) (6.6731, -50.9814) (6.5463, -51.3527) knots 0 0 0 0 0.08497 0.202683 0.202683 0.202683 0.202683
  spline S45 degree 3 poles (7.7578, -51.2053) (7.6435, -50.8598) (7.4481, -50.2692) (7.262, -49.6755) (7.1848, -49.4291) knots 0 0 0 0 0.109171 0.186642 0.186642 0.186642 0.186642
  line L19 (10.5981, -59.7019) -> (7.7578, -51.2053)
  line L20 (12.9883, -59.7019) -> (10.5981, -59.7019)
  line L21 (12.9883, -47.7019) -> (12.9883, -59.7019)
  line L22 (16.0209, -47.7019) -> (24.9759, -47.7019)
  line L23 (16.0209, -49.118) -> (16.0209, -47.7019)
  line L24 (23.3879, -49.118) -> (16.0209, -49.118)
  line L25 (23.3879, -53.2026) -> (23.3879, -49.118)
  line L26 (16.7494, -53.2026) -> (23.3879, -53.2026)
  line L27 (16.7494, -54.6105) -> (16.7494, -53.2026)
  line L28 (23.3879, -54.6105) -> (16.7494, -54.6105)
  line L29 (23.3879, -58.2858) -> (23.3879, -54.6105)
  line L30 (16.2992, -58.2858) -> (23.3879, -58.2858)
  line L31 (16.2992, -59.7019) -> (16.2992, -58.2858)
  line L32 (24.9759, -59.7019) -> (16.2992, -59.7019)
  line L33 (24.9759, -47.7019) -> (24.9759, -59.7019)
extrude "Extrude6" cut sketch "sketch 946" against normal blind 0.2 bodies 1
equation "d128 = -clearance"
equation "clearance = 0.2 mm"

design "FPA_Trapezoidal Nut"
Autodesk Fusion 360 part; units mm, degrees